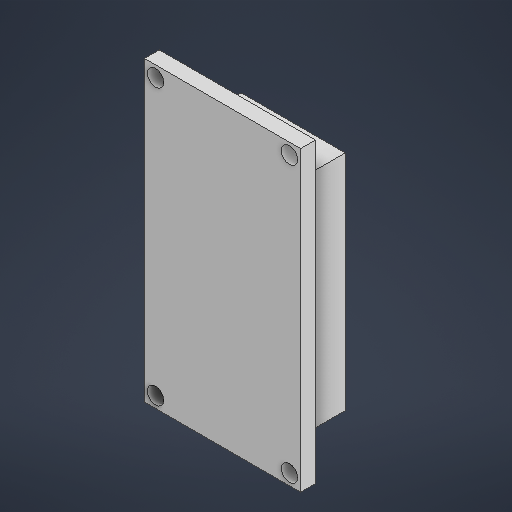
# Autodesk Inventor part: 7_Seg_Display_TM1637
Saved by Autodesk Inventor 2026.2 (Build 302298000, 298)
## iProperties
Created: 2026-03-17
Part Number: 7_Seg_Display_TM1637
Material: Generic
Document SubType Name: Modeling
Designer: vckot
Density: 1 g/cm^3
Appearance: Default
Author: vckot
Autodesk Inventor part; units mm, degrees
ref_plane "YZ Plane" through (0, 0, 0) normal (1, 0, 0) x (0, 1, 0)
ref_plane "XZ Plane" through (0, 0, 0) normal (0, 1, 0) x (-1, 0, 0)
ref_plane "XY Plane" through (0, 0, 0) normal (0, 0, 1) x (1, 0, 0)
sketch "Sketch1" plane through (0, 0, 0) normal (0, 1, 0) x (-1, 0, 0)
  line L0 (-10.5, 20) -> (10.5, 20)
  line L1 (10.5, 20) -> (10.5, -20)
  line L2 (10.5, -20) -> (-10.5, -20)
  line L3 (-10.5, -20) -> (-10.5, 20)
  line L4 (-10.5, 20) -> (10.5, -20) construction
  line L5 (10.5, 20) -> (-10.5, -20) construction
  point P0 (0, 0)
  dimension "d0" = 40
  dimension "d1" = 21
  constraints: 12 end point, 2 midpoint, 2 parallel, 1 horizontal, 1 perpendicular
  measures "d0" distance of L0.end L1.end
  measures "d1" distance of L1.end L2.end
extrude "Extrusion1" add sketch "Sketch1" along normal blind 2
sketch "Sketch2" plane through (0, 2, 0) normal (0, 1, 0) x (1, 0, 0)
  line L0 (-10.5, 20) -> (-10.5, -20) projected
  line L1 (-10.5, -20) -> (10.5, -20) projected
  line L2 (10.5, -20) -> (10.5, 20) projected
  line L3 (10.5, 20) -> (-10.5, 20) projected
  point P0 (0, 0)
  point P1 (-9, -18.5)
  point P2 (-9, 18.5)
  point P3 (9, 18.5)
  point P4 (9, -18.5)
  dimension "d4" = 1.5
  dimension "d5" = 1.5
  dimension "d6" = 1.5
  dimension "d7" = 1.5
  dimension "d20" = 18
  dimension "d21" = 18
  dimension "d22" = 37
  constraints: 2 horizontal alignment, 2 vertical alignment
  measures "d4" distance from line of L0 point (-9, -18.5)
  measures "d5" distance from line of L1 point (-9, -18.5)
  measures "d6" distance from line of L2 point (9, -18.5)
  measures "d7" distance from line of L3 point (-9, 18.5)
  measures "d20" distance of point (9, 18.5) point (-9, 18.5)
  measures "d21" distance of point (9, -18.5) point (-9, -18.5)
  measures "d22" distance of point (-9, 18.5) point (-9, -18.5)
hole "Hole1" at (-9, 2, 18.5) at (-9, 2, -18.5) at (9, 2, -18.5) at (9, 2, 18.5) direction (0, -1, 0) diameter 2.2 end through all
sketch "Sketch3" plane through (0, 2, 0) normal (0, 1, 0) x (1, 0, 0)
  line L0 (7.5, -13.5) -> (-6.5, -13.5)
  line L1 (-6.5, -13.5) -> (-6.5, 16.5)
  line L2 (-6.5, 16.5) -> (7.5, 16.5)
  line L3 (7.5, 16.5) -> (7.5, -13.5)
  line L4 (7.5, -13.5) -> (-6.5, 16.5) construction
  line L5 (-6.5, -13.5) -> (7.5, 16.5) construction
  line L6 (-10.5, -20) -> (10.5, -20) projected
  line L7 (-10.5, 20) -> (-10.5, -20) projected
  line L8 (10.5, 20) -> (-10.5, 20) projected
  point P0 (0, 0)
  point P1 (0.5, 1.5)
  point P2 (0, -20)
  dimension "d15" = 6.5
  dimension "d16" = 30
  dimension "d17" = 14
  dimension "d18" = 4
  dimension "d19" = 3.5
  constraints: 12 end point, 3 midpoint, 2 parallel, 1 horizontal, 1 perpendicular
  measures "d15" distance from line of point (0, -20) L0
  measures "d16" distance of L0.end L1.end
  measures "d17" distance of L1.end L2.end
  measures "d18" distance between parallel lines of L7 L1
  measures "d19" distance between parallel lines of L8 L2
extrude "Extrusion2" add sketch "Sketch3" along normal blind 7
body "Solid1"
